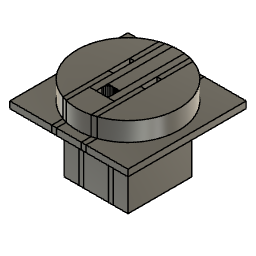
plug_3_pin_hole (Autodesk Fusion 360 design; units mm, degrees)
Autodesk Fusion 360 part; units mm, degrees
note: some values were not read from the file. Chosen so that the rebuilt part matches the saved one: which bodies a step acts on.
sketch "Sketch1" plane through (0, 0, 0) normal (0, 0, 1) x (1, 0, 0)
  line L0 (25, -25) -> (-25, -25)
  line L1 (-25, -25) -> (-25, 25)
  line L2 (-25, 25) -> (25, 25)
  line L3 (25, 25) -> (25, -25)
  line L4 (25, -25) -> (-25, 25) construction
  line L5 (-25, -25) -> (25, 25) construction
  dimension "d1" = 50
  dimension "d2" = 50
  constraint horizontal L0
  constraint perpendicular L0 L1
  constraint parallel L0 L2
  constraint parallel L1 L3
  constraint coincident L4 origin
  constraint coincident L5 origin
  measures "d1" distance of L1.end L2.end
  measures "d2" distance of L0.start L2.end
extrude "Extrude1" add sketch "Sketch1" against normal blind 2.8 makes body 1
sketch "Sketch2" plane through (0, 0, 0) normal (0, 0, 1) x (-1, 0, 0)
  line L0 (-25, -25) -> (25, -25)
  line L1 (25, -25) -> (25, 25)
  line L2 (25, 25) -> (-25, 25)
  line L3 (-25, 25) -> (-25, -25)
  circle A0 centre (0, 0) radius 21.5
  dimension "d5" = 43
  constraint coincident A0.centre origin
  measures "d5" diameter of A0
extrude "Extrude2" add sketch "Sketch2" along normal blind 8 contours A0 bodies 1
sketch "Sketch3" plane through (0, 0, 8) normal (0, 0, 1) x (-1, 0, 0)
  circle A0 centre (0, 0) radius 21.5
  line L0 (7.25, -8) -> (5.25, -8)
  line L1 (5.25, -8) -> (5.25, 1)
  line L2 (5.25, 1) -> (7.25, 1)
  line L3 (7.25, 1) -> (7.25, -8)
  line L4 (-5.25, -7) -> (-7.25, -7)
  line L5 (-7.25, -7) -> (-7.25, 0)
  line L6 (-7.25, 0) -> (-5.25, 0)
  line L7 (-5.25, 0) -> (-5.25, -7)
  line L8 (-2.5, 8.5) -> (-2.5, 11)
  line L9 (-2.5, 11) -> (2.5, 11)
  line L10 (2.5, 11) -> (2.5, 8.5)
  arc A1 (-2.5, 8.5) -> (2.5, 8.5) centre (0, 8.5) ccw
  dimension "d8" = 9
  dimension "d9" = 2
  dimension "d10" = 7
  dimension "d11" = 2
  dimension "d12" = 5
  dimension "d13" = 5
  dimension "d14" = 2.5
  dimension "d15" = 10.5
  dimension "d16" = 1
  dimension "d17" = 11
  dimension "d18" = 2.75
  constraint horizontal L0
  constraint vertical L1
  constraint horizontal L2
  constraint vertical L3
  constraint horizontal L4
  constraint vertical L5
  constraint horizontal L6
  constraint vertical L7
  constraint vertical L8
  constraint horizontal L9
  constraint vertical L10
  constraint vertical A0.centre A1.centre
  constraint coincident A0.centre L6
  measures "d8" distance of L0.end L1.end
  measures "d9" distance of L0.start L0.end
  measures "d10" distance of L4.end L5.end
  measures "d11" distance of L4.start L4.end
  measures "d12" diameter of A1
  measures "d13" distance of L10.end L8.start
  measures "d14" distance of L10.end L9.end
  measures "d15" distance of L1 L7
  measures "d16" distance of L0 L4
  measures "d17" distance of L6 L9
  measures "d18" distance of L7 L8
extrude "Extrude3" cut sketch "Sketch3" against normal blind 21 contours L0 L1 L2 L3 | L4 L5 L6 L7 | L8 L9 L10 A1 bodies 1
sketch "Sketch4" plane through (0, 0, -2.8) normal (0, 0, -1) x (1, 0, 0)
  line L0 (-5.25, 1) -> (-5.25, -8)
  line L1 (-5.25, -8) -> (-7.25, -8)
  line L2 (-7.25, -8) -> (-7.25, 1)
  line L3 (-7.25, 1) -> (-5.25, 1)
  line L4 (7.25, 0) -> (7.25, -7)
  line L5 (7.25, -7) -> (5.25, -7)
  line L6 (5.25, -7) -> (5.25, 0)
  line L7 (5.25, 0) -> (7.25, 0)
  arc A0 (-2.5, 8.5) -> (2.5, 8.5) centre (0, 8.5) ccw
  line L8 (-2.5, 8.5) -> (-2.5, 11)
  line L9 (-2.5, 11) -> (2.5, 11)
  line L10 (2.5, 11) -> (2.5, 8.5)
  line L11 (-25, -25) -> (25, -25)
  line L12 (25, -25) -> (25, 25)
  line L13 (25, 25) -> (-25, 25)
  line L14 (-25, 25) -> (-25, -25)
  line L15 (13.5, -13.5) -> (-13.5, -13.5)
  line L16 (-13.5, -13.5) -> (-13.5, 13.5)
  line L17 (-13.5, 13.5) -> (13.5, 13.5)
  line L18 (13.5, 13.5) -> (13.5, -13.5)
  line L19 (13.5, -13.5) -> (-13.5, 13.5) construction
  line L20 (-13.5, -13.5) -> (13.5, 13.5) construction
  dimension "d21" = 27
  dimension "d22" = 27
  constraint horizontal L15
  constraint perpendicular L15 L16
  constraint parallel L15 L17
  constraint parallel L16 L18
  constraint coincident L19 origin
  constraint coincident L20 origin
  measures "d21" distance of L16.end L17.end
  measures "d22" distance of L15.end L16.end
extrude "Extrude4" add sketch "Sketch4" along normal blind 25 contours L15 L16 L17 L18 bodies 1
move_body "Move1" bodies 1 to x (1, 0, 0) y (0, 1, 0) z (0, 0, 1) at (0, 0, 27.8)
move_body "Move2" bodies 1 to x (1, 0, 0) y (0, 1, 0) z (0, 0, 1) at (-13.5, 13.5, 0)
move_body "Move3" bodies 1 to x (1, 0, 0) y (0, 1, 0) z (0, 0, 1) at (13.5, -13.5, 0)
split "Split1" by plane through (-7.25, 8, 25) normal (1, 0, 0) bodies 1 makes body 2 at (21.1667, -4.5, 25)
split "Split2" by plane through (-5.25, -1, 25) normal (-1, 0, 0) bodies 2 makes body 3 at (-7.25, -5.1667, 20.2667) makes body 4 at (-7.25, 13.9136, 32.2)
split "Split3" by plane through (7.25, 0, 25) normal (-1, 0, 0) bodies 2 makes body 5 at (-5.25, -5.1667, 20.2667)
split "Split4" by plane through (5.25, 7, 25) normal (1, 0, 0) bodies 5 makes body 6 at (7.25, -4.5, 20.2667) makes body 7 at (7.25, 13.5802, 32.2)
split "Split5" by plane through (-2.5, -11, 25) normal (0, 1, 0) bodies 5 makes body 8 at (5.25, -3.6667, 23.8667)
split "Split6" by plane through (2.5, -11, 25) normal (-1, 0, 0) and through (-2.5, -8.5, 25) normal (1, 0, 0) bodies 8 makes body 9 at (-5.25, -7.6667, 23.8667) makes body 10 at (-2.1332, -7.1964, 23.8667)
ref_plane "WorkPlane1" through (-2.5, -8.5, 35.8) normal (0, 1, 0) x (-1, 0, 0)
ref_plane "WorkPlane2" through (0, -6, 31.1141) normal (0, -1, 0) x (1, 0, 0)
ref_plane "WorkPlane3" through (0, -5, 31.1141) normal (0, -1, 0) x (1, 0, 0)
split "Split7" by plane through (0, -5, 31.1141) normal (0, -1, 0) bodies 10 makes body 11 at (-2.1332, -7.1964, 23.8667)
ref_plane "WorkPlane4" through (0, -6.75, 17.9) normal (1, 0, 0) x (0, -1, 0)
split "Split8" by plane through (0, -6.75, 17.9) normal (1, 0, 0) bodies 11 makes body 12 at (2.4972, -8.381, 11.9333)
split "Split9" by plane through (0, -6, 31.1141) normal (0, -1, 0) bodies 12 makes body 13 at (2.4972, -8.381, 11.9333)
split "Split10" by plane through (0, -6, 31.1141) normal (0, -1, 0) bodies 11 makes body 14 at (-2.4887, -8.2624, 23.8667)
combine "Combine1" operation add target body 10 tool bodies 11 12
ref_plane "WorkPlane5" through (0, -8.5, 17.9) normal (0.258819, 0.965926, 0) x (0, 0, -1)
ref_plane "WorkPlane6" through (0, -8.5, 17.9) normal (0.5, 0.866025, 0) x (0, 0, -1)
ref_plane "WorkPlane7" through (0, -8.5, 17.9) normal (0.707107, 0.707107, 0) x (0, 0, -1)
ref_plane "WorkPlane8" through (0, -8.5, 17.9) normal (0.866025, 0.5, 0) x (0, 0, -1)
ref_plane "WorkPlane9" through (0, -8.5, 17.9) normal (0.866025, 0.5, 0) x (0, 0, -1)
ref_plane "WorkPlane10" through (0, -8.5, 17.9) normal (0.965926, 0.258819, 0) x (0, 0, -1)
ref_plane "WorkPlane11" through (0, -8.5, 17.9) normal (0.965926, -0.258819, 0) x (0, 0, -1)
ref_plane "WorkPlane12" through (0, -8.5, 17.9) normal (0.866025, -0.5, 0) x (0, 0, -1)
ref_plane "WorkPlane13" through (0, -8.5, 17.9) normal (0.707107, -0.707107, 0) x (0, 0, -1)
ref_plane "WorkPlane14" through (0, -8.5, 17.9) normal (0.5, -0.866025, 0) x (0, 0, -1)
ref_plane "WorkPlane15" through (0, -8.5, 17.9) normal (0.258819, -0.965926, 0) x (0, 0, -1)
split "Split11" by plane through (0, -8.5, 17.9) normal (0.258819, 0.965926, 0) bodies 14 makes body 15 at (-1.835, -6.8021, 23.8667)
split "Split12" by plane through (0, -8.5, 17.9) normal (0.5, 0.866025, 0) bodies 15 makes body 16 at (-0.2489, -6.0124, 11.9333)
split "Split13" by plane through (0, -8.5, 17.9) normal (0.707107, 0.707107, 0) bodies 16 makes body 17 at (-0.8333, -6, 23.8667)
split "Split14" by plane through (0, -8.5, 17.9) normal (0.866025, 0.5, 0) bodies 17 makes body 18 at (-0.9623, -6, 23.8667)
split "Split15" by plane through (0, -8.5, 17.9) normal (0.965926, 0.258819, 0) bodies 18 makes body 19 at (-0.2233, -6, 11.9333)
split "Split16" by plane through (0, -8.5, 17.9) normal (0.965926, -0.258819, 0) bodies 13 makes body 20 at (2.0197, -7.0266, 11.9333)
split "Split17" by plane through (0, -8.5, 17.9) normal (0.866025, -0.5, 0) bodies 20 makes body 21 at (2.4876, -8.2511, 23.8667)
split "Split18" by plane through (0, -8.5, 17.9) normal (0.707107, -0.707107, 0) bodies 21 makes body 22 at (2.5, -6.8333, 23.8667)
split "Split19" by plane through (0, -8.5, 17.9) normal (0.5, -0.866025, 0) bodies 22 makes body 23 at (2.5, -7.5377, 11.9333)
split "Split20" by plane through (0, -8.5, 17.9) normal (0.258819, -0.965926, 0) bodies 23 makes body 24 at (2.5, -8.0534, 11.9333)
move_body "Move4" bodies 2 7 1 18 9 16 21 3 8 20 15 5 22 23 10 14 6 17 24 19 4 13 to x (1, 0, 0) y (0, 1, 0) z (0, 0, 1) at (0, 0, -36)
named bodies: "Body11", "Body12", "Body13", "Body14", "Body15", "Body16", "Body17", "Body18", "Body19", "Body20", "Body21", "Body22"
